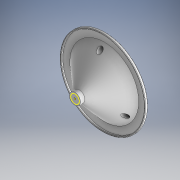
# Autodesk Inventor part: meteostanica lievik
Saved by Autodesk Inventor 2017.3 (Build 213256000, 256)
## iProperties
Created: 2017-02-23
Part Number: meteostanica lievik
Material: ABS Plastic
Document SubType Name: Modeling
Designer: Luc3as
Density: 1.06 g/cm^3
Appearance: Smooth - White
Author: Luc3as
Autodesk Inventor part; units mm, degrees
ref_plane "YZ Plane" through (0, 0, 0) normal (1, 0, 0) x (0, 1, 0)
ref_plane "XZ Plane" through (0, 0, 0) normal (0, 1, 0) x (-1, 0, 0)
ref_plane "XY Plane" through (0, 0, 0) normal (0, 0, 1) x (1, 0, 0)
sketch "Sketch1" plane through (0, 0, 0) normal (0, 1, 0) x (-1, 0, 0)
  circle A0 centre (0, 0) radius 48
  circle A1 centre (0, 0) radius 41
  circle A2 centre (0, 0) radius 26
  line L0 (0, 41) -> (0, 34)
  circle A3 centre (0, 34) radius 3
  circle A4 centre (29.4449, -17) radius 3
  circle A5 centre (-29.4449, -17) radius 3
  dimension "d2" = 82
  dimension "d0" = 96
  dimension "d53" = 15
  dimension "d54" = 7
  dimension "d55" = 6
  dimension "d56" = 6
  dimension "d57" = 6
  constraints: 5 centre point, 4 coincident, 2 end point, 1 vertical, 1 vertical alignment, 2 other
  measures "d0" diameter of A0
  measures "d54" distance of L0.start L0.end
  measures "d55" diameter of A3
  measures "d56" diameter of A4
  measures "d57" diameter of A5
extrude "Extrusion1" add sketch "Sketch1" against normal blind 30 contours A1 | A2 | A3 | A4 | A5
sketch "Sketch4" plane through (0, -30, 0) normal (0, -1, 0) x (1, 0, 0)
  circle A0 centre (0, 0) radius 5
  dimension "d6" = 10
  constraints: 1 centre point, 1 coincident
  measures "d6" diameter of A0
extrude "Extrusion2" cut sketch "Sketch4" against normal blind 30
draft "FaceDraft1" angle 49 pull direction (0, -1, 0) faces at (17.8845, -10, 36.8937) fixed edges at (41, 0, 0)
draft "FaceDraft2" angle 49 pull direction (0, 1, 0) faces at (4.9838, -10, -0.4023) fixed edges at (-5, -30, 0)
sketch "Sketch5" plane through (0, -30, 0) normal (0, -1, 0) x (1, 0, 0)
  circle A0 centre (0, 0) radius 5 projected
  circle A1 centre (0, 0) radius 6.4889 projected
extrude "Extrusion3" add sketch "Sketch5" along normal blind 5
sketch "Sketch6" plane through (0, 0, 0) normal (0, 1, 0) x (1, 0, 0)
  circle A0 centre (0, 0) radius 48
  circle A1 centre (0, 0) radius 39.5111 projected
  dimension "d13" = 96
  constraints: 1 centre point, 1 coincident
  measures "d13" diameter of A0
extrude "Extrusion4" add sketch "Sketch6" against normal blind 1
sketch "Sketch9" plane through (0, 0, 0) normal (0, 1, 0) x (1, 0, 0)
  circle A0 centre (0, 0) radius 48 projected
  circle A1 centre (0, 0) radius 49.5
  dimension "d20" = 1.5
  constraints: 1 centre point
  measures "d20" radial gap between concentric circles of A0 A1
extrude "Extrusion6" add sketch "Sketch9" against normal blind 3
fillet "Fillet1" radius 0.5 2 edges at (-48, -3, 0) (-49.5, -3, 0)
fillet "Fillet2" radius 0.5 1 edges at (-49.5, 0, 0)
fillet "Fillet3" radius 2 1 edges at (-39.5111, 0, 0)
sketch "Sketch10" plane through (0, 0, 0) normal (0, 1, 0) x (1, 0, 0)
  line L0 (-27.9992, 29.1572) -> (29.2485, -28.0289)
  line L1 (-29.7576, 27.3987) -> (27.3516, -29.9257)
  line L2 (29.6539, 27.3123) -> (-27.3516, -29.9257)
  line L3 (27.9093, 29.0569) -> (-29.2485, -28.0289)
  line L4 (-27.9992, 29.1572) -> (-29.7576, 27.3987)
  line L5 (29.2485, -28.0289) -> (27.3516, -29.9257)
  line L6 (-29.2485, -28.0289) -> (-27.3516, -29.9257)
  line L7 (27.9093, 29.0569) -> (29.6539, 27.3123)
  line L8 (-10.9187, 39.5619) -> (39.967, -11.3238)
  line L9 (-39.7995, 10.1025) -> (10.1276, -39.8247)
  line L10 (10.6928, 39.2349) -> (-39.5283, -10.9862)
  line L11 (39.724, 10.0325) -> (-10.0559, -39.7474)
  line L12 (8.5418, 39.9123) -> (-40.138, -8.7674)
  line L13 (40.3337, 7.8137) -> (-8.1927, -40.7127)
  line L14 (-40.161, 7.6355) -> (7.9089, -40.4343)
  line L15 (-9.3567, 40.8283) -> (41.3812, -9.9096)
  line L16 (41.3812, -9.9096) -> (39.967, -11.3238)
  line L17 (39.724, 10.0325) -> (40.3337, 7.8137)
  line L18 (8.5418, 39.9123) -> (10.6928, 39.2349)
  line L19 (-9.3567, 40.8283) -> (-10.9187, 39.5619)
  line L20 (-39.7995, 10.1025) -> (-40.161, 7.6355)
  line L21 (-40.138, -8.7674) -> (-39.5283, -10.9862)
  line L22 (-10.0559, -39.7474) -> (-8.1927, -40.7127)
  line L23 (7.9089, -40.4343) -> (10.1276, -39.8247)
  point P0 (0, 0)
  dimension "d45" = 20
  dimension "d46" = 20
  dimension "d47" = 20
  dimension "d48" = 20
  dimension "d49" = 2
  dimension "d50" = 2
  dimension "d51" = 2
  dimension "d52" = 2
  constraints: 48 end point, 5 parallel, 1 perpendicular
  measures "d45" distance of L0.start L8.start
  measures "d46" distance of L1.start L9.start
  measures "d47" distance of L3.start L10.start
  measures "d48" distance of L2.start L11.start
  measures "d49" distance between parallel lines of L10 L12
  measures "d50" distance between parallel lines of L11 L13
  measures "d51" distance between parallel lines of L9 L14
  measures "d52" distance between parallel lines of L8 L15
extrude "Extrusion7" add sketch "Sketch10" against normal blind 1 contours L0 L12 L1 L4 | L12 L8 L10 L0 | L0 L10 L1 L12 | L0 L3 L1 L10 | L12 L15 L10 L8 | L8 L19 L15 L12 | L1 L10 L9 L12 | L3 L8 L2 L0 | L0 L2 L1 L3 | L10 L15 L3 L8 | L12 L18 L10 L15 | L12 L14 L20 L9 | L9 L10 L14 L12 | L0 L11 L1 L2 | L3 L15 L2 L8 | L1 L2 L9 L3 | L9 L3 L14 L10 | L14 L10 L21 L12 | L11 L8 L13 L0 | L0 L13 L1 L11 | L2 L15 L11 L8 | L3 L7 L2 L15 | L9 L2 L14 L3 | L0 L5 L1 L13 | L11 L15 L13 L8 | L1 L13 L9 L11 | L9 L11 L14 L2 | L14 L2 L6 L3 | L13 L15 L16 L8 | L11 L17 L13 L15 | L9 L13 L14 L11 | L9 L23 L14 L13 | L14 L13 L22 L11
sketch "Sketch11" plane through (0, 0, 0) normal (0, 1, 0) x (1, 0, 0)
  circle A0 centre (0, 0) radius 41
  line L0 (0, -41) -> (0, -34)
  circle A1 centre (0, -34) radius 3
  circle A2 centre (29.4449, 17) radius 3
  circle A3 centre (-29.4449, 17) radius 3
  circle A4 centre (29.4449, 17) radius 5
  circle A5 centre (0, -34) radius 5
  circle A6 centre (-29.4449, 17) radius 5
  dimension "d58" = 82
  dimension "d60" = 7
  dimension "d61" = 6
  dimension "d62" = 6
  dimension "d63" = 6
  dimension "d64" = 2
  dimension "d65" = 2
  dimension "d66" = 2
  constraints: 6 centre point, 3 coincident, 2 end point, 1 vertical, 1 vertical alignment, 2 other
  measures "d60" distance of L0.start L0.end
  measures "d61" diameter of A1
  measures "d62" diameter of A2
  measures "d63" diameter of A3
  measures "d64" radial gap between concentric circles of A2 A4
  measures "d65" radial gap between concentric circles of A1 A5
  measures "d66" radial gap between concentric circles of A3 A6
extrude "Extrusion8" add sketch "Sketch11" against normal through all contours A1 | A2 | A3 | A4 | A5 | A6
hole "Hole1" at (29.4449, 0, -17) direction (0, -1, 0) diameter 6 end through all
hole "Hole2" at (0, 0, 34) at (-29.4449, 0, -17) direction (0, -1, 0) diameter 6 end through all
sketch "Sketch12" plane through (0, -35, 0) normal (0, -1, 0) x (1, 0, 0)
  circle A0 centre (0, 0) radius 5 projected
extrude "Extrusion9" add sketch "Sketch12" against normal blind 5
sketch "Sketch13" plane through (0, -30, 0) normal (0, 1, 0) x (1, 0, 0)
  circle A0 centre (0, 0) radius 5 projected
  circle A1 centre (0, -34) radius 3 projected
  arc A2 (-2.7206, -29.8049) -> (-4.9577, -34.6492) centre (0, -34) ccw projected
  line L0 (-4.9577, -34.6492) -> (-9.444, -39.1355) projected
  arc A3 (-27.1516, -29.7248) -> (-9.444, -39.1355) centre (0, 0) ccw projected
  line L1 (-15.0009, -17.5246) -> (-27.1516, -29.7248) projected
  line L2 (-2.7206, -29.8049) -> (-15.0009, -17.5246) projected
  line L3 (-13.5896, -16.1075) -> (-0.6541, -29.043) projected
  line L4 (-0.0042, -2.4668) -> (-13.5896, -16.1075) projected
  line L5 (13.5847, -16.1069) -> (-0.0042, -2.4668) projected
  line L6 (13.5847, -16.1069) -> (0.6492, -29.0423) projected
  arc A4 (0.6492, -29.0423) -> (-0.6541, -29.043) centre (0, -34) ccw projected
  line L7 (2.7172, -29.8027) -> (14.9962, -17.5237) projected
  line L8 (27.1515, -29.7249) -> (14.9962, -17.5237) projected
  arc A5 (9.4395, -39.1365) -> (27.1515, -29.7249) centre (0, 0) ccw projected
  line L9 (4.957, -34.6541) -> (9.4395, -39.1365) projected
  arc A6 (4.957, -34.6541) -> (2.7172, -29.8027) centre (0, -34) ccw projected
  circle A7 centre (0, 0) radius 49 projected
  line L10 (0.0505, 28.5926) -> (13.7389, 14.9043) projected
  line L11 (0.0027, 1.1855) -> (13.7389, 14.9043) projected
  line L12 (-13.6843, 14.8578) -> (0.0027, 1.1855) projected
  line L13 (0.0505, 28.5926) -> (-13.6843, 14.8578) projected
  line L14 (29.1673, -0.5242) -> (15.4481, -14.2434) projected
  line L15 (1.8226, -0.6325) -> (15.4481, -14.2434) projected
  line L16 (15.5212, 13.122) -> (1.8226, -0.6325) projected
  line L17 (15.5212, 13.122) -> (29.1673, -0.5242) projected
  line L18 (-15.4774, 13.0647) -> (-29.1196, -0.5775) projected
  line L19 (-1.8246, -0.6395) -> (-15.4774, 13.0647) projected
  line L20 (-15.4497, -14.2474) -> (-1.8246, -0.6395) projected
  line L21 (-29.1196, -0.5775) -> (-15.4497, -14.2474) projected
  line L22 (-16.889, 14.4816) -> (-29.6225, 27.2631) projected
  line L23 (-30.5338, 0.8367) -> (-16.889, 14.4816) projected
  line L24 (-39.1365, 9.4395) -> (-30.5338, 0.8367) projected
  arc A8 (-29.6225, 27.2631) -> (-39.1365, 9.4395) centre (0, 0) ccw projected
  line L25 (15.154, 16.3176) -> (27.8877, 29.0353) projected
  line L26 (15.154, 16.3176) -> (1.4647, 30.0068) projected
  line L27 (10.3607, 38.9028) -> (1.4647, 30.0068) projected
  arc A9 (27.8877, 29.0353) -> (10.3607, 38.9028) centre (0, 0) ccw projected
  arc A10 (-39.6274, 7.102) -> (-39.4415, -8.071) centre (0, 0) ccw projected
  line L28 (-31.948, -0.5775) -> (-39.6274, 7.102) projected
  line L29 (-39.4415, -8.071) -> (-31.948, -0.5775) projected
  line L30 (39.4586, -7.987) -> (31.9958, -0.5242) projected
  line L31 (31.9958, -0.5242) -> (39.6266, 7.1067) projected
  arc A11 (39.4586, -7.987) -> (39.6266, 7.1067) centre (0, 0) ccw projected
  line L32 (16.8631, -15.6568) -> (29.0705, -27.851) projected
  line L33 (16.8631, -15.6568) -> (30.5816, -1.9384) projected
  line L34 (30.5816, -1.9384) -> (38.924, -10.2808) projected
  arc A12 (29.0705, -27.851) -> (38.924, -10.2808) centre (0, 0) ccw projected
  arc A13 (8.071, 39.4415) -> (-7.987, 39.4586) centre (0, 0) ccw projected
  line L35 (0.0505, 31.4211) -> (8.071, 39.4415) projected
  line L36 (0.0505, 31.4211) -> (-7.987, 39.4586) projected
  arc A14 (-38.9028, -10.3607) -> (-29.0705, -27.851) centre (0, 0) ccw projected
  line L37 (-30.5338, -1.9917) -> (-38.9028, -10.3607) projected
  line L38 (-16.8648, -15.6607) -> (-30.5338, -1.9917) projected
  line L39 (-29.0705, -27.851) -> (-16.8648, -15.6607) projected
  arc A15 (39.1355, 9.444) -> (29.614, 27.2723) centre (0, 0) ccw projected
  line L40 (39.1355, 9.444) -> (30.5816, 0.89) projected
  line L41 (30.5816, 0.89) -> (16.9325, 14.5391) projected
  line L42 (29.614, 27.2723) -> (16.9325, 14.5391) projected
  arc A16 (-10.2808, 38.924) -> (-27.8823, 29.0405) centre (0, 0) ccw projected
  line L43 (-10.2808, 38.924) -> (-1.3637, 30.0068) projected
  line L44 (-15.0993, 16.2712) -> (-1.3637, 30.0068) projected
  line L45 (-27.8823, 29.0405) -> (-15.0993, 16.2712) projected
  line L46 (7.102, -39.6274) -> (4.1951, -36.7206) projected
  arc A17 (-7.1067, -39.6266) -> (7.102, -39.6274) centre (0, 0) ccw projected
  line L47 (-7.1067, -39.6266) -> (-4.1973, -36.7172) projected
  arc A18 (-4.1973, -36.7172) -> (4.1951, -36.7206) centre (0, -34) ccw projected
  circle A19 centre (0, 0) radius 5 projected
hole "Hole3" at (0, -30, 0) direction (0, -1, 0) diameter 2 end through all countersink diameter 10 countersink angle 90
equation "\"d64\" = d66"
equation "\"d65\" = d66"
body "Solid1"
